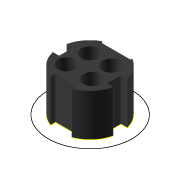
# Autodesk Inventor part: 00_Kycon_4pin_mail
Saved by Autodesk Inventor 2019.4 (Build 234330000, 330)
## iProperties
Created: 2020-10-06
Part Number: 00_Kycon_4pin_mail
Material: Generic
Document SubType Name: Modeling
Designer: diederichbenedict
Density: 1 g/cm^3
Appearance: Default
Author: diederichbenedict
Autodesk Inventor part; units mm, degrees
ref_plane "YZ Plane" through (0, 0, 0) normal (1, 0, 0) x (0, 1, 0)
ref_plane "XZ Plane" through (0, 0, 0) normal (0, 1, 0) x (-1, 0, 0)
ref_plane "XY Plane" through (0, 0, 0) normal (0, 0, 1) x (1, 0, 0)
sketch "Sketch1" plane through (0, 0, 0) normal (0, 1, 0) x (-1, 0, 0)
  circle A0 centre (0, 0) radius 4.375
  circle A1 centre (1.8, 1.5) radius 1.25
  circle A2 centre (1.5, -1.5) radius 1.25
  circle A3 centre (-1.8, 1.5) radius 1.25
  circle A4 centre (-1.5, -1.5) radius 1.25
  line L0 (1.4885, 4.7346) -> (0.1984, 4.7346)
  line L1 (-1.5115, 4.1056) -> (-1.5115, 3.4074)
  line L2 (-1.5115, 3.4074) -> (1.4885, 3.4074)
  line L3 (1.4885, 3.4074) -> (1.4885, 4.7346)
  line L4 (1.4885, 4.7346) -> (-1.5115, 3.4074) construction
  line L5 (0.1984, 4.7346) -> (1.4885, 3.4074) construction
  line L6 (2.1288, -3.5803) -> (-2.1422, -3.5803)
  line L7 (-2.1422, -3.5803) -> (-2.1422, -3.8146)
  line L8 (-2.1708, -5.1794) -> (2.1288, -5.1794)
  line L9 (2.1288, -5.1794) -> (2.1288, -3.5803)
  line L10 (4.2592, 1) -> (3.375, 1)
  line L11 (3.375, 1) -> (3.375, -1)
  line L12 (3.375, -1) -> (5.375, -1)
  line L13 (5.375, -1) -> (5.375, 1)
  line L14 (5.375, 1) -> (3.375, -1) construction
  line L15 (3.375, 1) -> (5.375, -1) construction
  line L16 (-3.375, 1) -> (-4.2592, 1)
  line L17 (-5.375, 1) -> (-5.375, -1)
  line L18 (-5.375, -1) -> (-3.375, -1)
  line L19 (-3.375, -1) -> (-3.375, 1)
  line L20 (-3.375, 1) -> (-5.375, -1) construction
  line L21 (-5.375, 1) -> (-3.375, -1) construction
  point P0 (0.5864, 4.3355)
  point P1 (0.2908, -4.3653)
  point P2 (1.4885, 4.114)
  point P3 (2.1288, -3.8221)
  point P4 (4.375, 0)
  point P5 (-4.375, 0)
  point P6 (-4.2592, -1)
  point P7 (4.2592, -1)
  dimension "d0" = 8.75
  dimension "d1" = 2.5
  dimension "d_1" = 2.5
  dimension "d3" = 2.5
  dimension "d4" = 2.5
  dimension "d5" = 1.5
  dimension "d6" = 1.5
  dimension "d7" = 1.5
  dimension "d8" = 1.5
  dimension "d9" = 1.8
  dimension "d10" = 1.8
  dimension "d11" = 1.5
  dimension "d12" = 1.5
  dimension "d13" = 3
  dimension "d19" = 2
  dimension "d20" = 2
  dimension "d21" = 2
  dimension "d22" = 2
  constraints: 44 end point, 8 parallel, 6 point on line, 4 centre point, 4 horizontal, 4 midpoint, 4 perpendicular, 1 coincident, 14 other
  measures "d1" diameter of A1
  measures "d_1" diameter of A2
  measures "d3" diameter of A3
  measures "d4" diameter of A4
  measures "d5" horizontal distance of A2.centre point (0, 0)
  measures "d6" horizontal distance of A4.centre point (0, 0)
  measures "d7" horizontal distance of point (0, 0) A2.centre
  measures "d8" horizontal distance of point (0, 0) A4.centre
  measures "d9" horizontal distance of point (0, 0) A1.centre
  measures "d10" horizontal distance of A3.centre point (0, 0)
  measures "d11" vertical distance of point (0, 0) A3.centre
  measures "d12" vertical distance of point (0, 0) A1.centre
  measures "d13" distance of L2.end L1.end
  measures "d19" distance of L12.end L11.end
  measures "d20" distance of L11.end L10.end
  measures "d21" distance of L18.end L17.end
  measures "d22" distance of L17.end L17.start
extrude "Extrusion1" add sketch "Sketch1" along normal blind 6 contours L10 L11 L12 A0 L9 L6 L7 L18 L19 L16 L1 L2 L3
sketch "Sketch2" plane through (0, 0, 0) normal (0, -1, 0) x (1, 0, 0)
  circle A0 centre (1.5, -1.5) radius 1.25 projected
  circle A1 centre (1.8, 1.5) radius 1.25 projected
  circle A2 centre (-1.5, -1.5) radius 1.25 projected
  circle A3 centre (-1.8, 1.5) radius 1.25 projected
  line L0 (1.5115, 3.4074) -> (1.5115, 4.1056) projected
  line L1 (-1.4885, 3.4074) -> (1.5115, 3.4074) projected
  line L2 (-1.4885, 4.114) -> (-1.4885, 3.4074) projected
  arc A4 (-1.4885, 4.114) -> (-4.2592, 1) centre (0, 0) ccw projected
  line L3 (-3.375, 1) -> (-4.2592, 1) projected
  line L4 (-3.375, -1) -> (-3.375, 1) projected
  line L5 (-4.2592, -1) -> (-3.375, -1) projected
  arc A5 (-4.2592, -1) -> (-2.1288, -3.8221) centre (0, 0) ccw projected
  line L6 (-2.1288, -3.5803) -> (-2.1288, -3.8221) projected
  line L7 (2.1422, -3.5803) -> (-2.1288, -3.5803) projected
  line L8 (2.1422, -3.8146) -> (2.1422, -3.5803) projected
  arc A6 (2.1422, -3.8146) -> (4.2592, -1) centre (0, 0) ccw projected
  line L9 (3.375, -1) -> (4.2592, -1) projected
  line L10 (3.375, 1) -> (3.375, -1) projected
  line L11 (4.2592, 1) -> (3.375, 1) projected
  arc A7 (4.2592, 1) -> (1.5115, 4.1056) centre (0, 0) ccw projected
  circle A8 centre (0, 0) radius 5.9296
  constraints: 1 centre point, 1 coincident
equation "\"d1\" = d_1"
equation "\"d3\" = d_1"
equation "\"d4\" = d_1"
body "Solid1"
